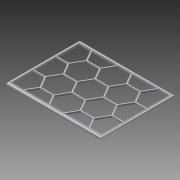
# Autodesk Inventor part: plate
Saved by Autodesk Inventor 2014 SP1 (Build 180222100, 222)
## iProperties
Created: 2016-09-05
Part Number: plate
Material: ABS Plastic
Document SubType Name: Modeling
Designer: tguillod
Density: 1.06 g/cm^3
Appearance: Smooth - White
Author: tguillod
Autodesk Inventor part; units mm, degrees
ref_plane "YZ Plane" through (0, 0, 0) normal (1, 0, 0) x (0, 1, 0)
ref_plane "XZ Plane" through (0, 0, 0) normal (0, 1, 0) x (-1, 0, 0)
ref_plane "XY Plane" through (0, 0, 0) normal (0, 0, 1) x (1, 0, 0)
sketch "Sketch1" plane through (0, 0, 0) normal (0, 0, 1) x (1, 0, 0)
  line L0 (0, 0) -> (183.5, 0)
  line L1 (183.5, 0) -> (183.5, 143)
  line L2 (183.5, 143) -> (0, 143)
  line L3 (0, 143) -> (0, 0)
  dimension "d0" = 183.5
  dimension "d1" = 143
  constraints: 8 end point, 2 parallel, 1 horizontal, 1 perpendicular
  measures "d0" distance of L1.end L2.end
  measures "d1" distance of L0.end L1.end
extrude "Extrusion1" add sketch "Sketch1" along normal blind 3
sketch "Sketch12" plane through (0, 0, 3) normal (0, 0, 1) x (1, 0, 0)
  line L0 (0, 0) -> (183.5, 0) projected
  line L1 (183.5, 0) -> (183.5, 143) projected
  line L2 (183.5, 143) -> (0, 143) projected
  line L3 (0, 143) -> (0, 0) projected
  line L4 (3, 5) -> (4, 5)
  line L5 (4, 5) -> (4, 140)
  line L6 (4, 140) -> (3, 140)
  line L7 (3, 140) -> (3, 5)
  line L8 (4, 140) -> (179.5, 140)
  line L9 (179.5, 140) -> (179.5, 139)
  line L10 (179.5, 139) -> (4, 139)
  line L11 (4, 139) -> (4, 140)
  line L12 (179.5, 140) -> (180.5, 140)
  line L13 (180.5, 140) -> (180.5, 5)
  line L14 (180.5, 5) -> (179.5, 5)
  line L15 (179.5, 5) -> (179.5, 140)
  dimension "d77" = 3
  dimension "d78" = 1
  dimension "d79" = 5
  dimension "d80" = 3
  dimension "d81" = 1
  dimension "d82" = 3
  dimension "d83" = 1
  constraints: 24 end point, 6 parallel, 3 horizontal, 3 perpendicular, 1 collinear
  measures "d77" distance between parallel lines of L3 L7
  measures "d78" distance of L4.start L4.end
  measures "d79" distance between parallel lines of L0 L4
  measures "d80" distance between parallel lines of L2 L8
  measures "d81" distance between parallel lines of L8 L10
  measures "d82" distance between parallel lines of L1 L13
  measures "d83" distance between parallel lines of L13 L15
extrude "Extrusion7" add sketch "Sketch12" along normal blind 1 contours L7 L6 L5 L4 | L5 L8 L9 L10 | L9 L12 L13 L14 L15
sketch "Sketch13" plane through (0, 0, 3) normal (0, 0, 1) x (1, 0, 0)
  line L0 (4, 139) -> (179.5, 139)
  line L1 (179.5, 139) -> (179.5, 5)
  line L2 (179.5, 5) -> (4, 5)
  line L3 (4, 5) -> (4, 139)
  line L4 (91.75, 139) -> (91.75, 5) construction
  line L5 (179.5, 72) -> (4, 72) construction
  line L6 (104.163, 50.5) -> (79.337, 50.5)
  line L7 (79.337, 50.5) -> (66.9239, 72)
  line L8 (66.9239, 72) -> (79.337, 93.5)
  line L9 (79.337, 93.5) -> (104.163, 93.5)
  line L10 (104.163, 93.5) -> (116.5761, 72)
  line L11 (116.5761, 72) -> (104.163, 50.5)
  line L12 (105.3177, 48.5) -> (78.1823, 48.5)
  line L13 (78.1823, 48.5) -> (64.6145, 72)
  line L14 (64.6145, 72) -> (78.1823, 95.5)
  line L15 (78.1823, 95.5) -> (105.3177, 95.5)
  line L16 (105.3177, 95.5) -> (118.8855, 72)
  line L17 (118.8855, 72) -> (105.3177, 48.5)
  line L18 (4, 139) -> (179.5, 139) projected
  line L19 (105.3177, 93.5) -> (78.1823, 93.5)
  line L20 (78.1823, 93.5) -> (64.6145, 117)
  line L21 (64.6145, 117) -> (78.1823, 140.5)
  line L22 (78.1823, 140.5) -> (105.3177, 140.5)
  line L23 (105.3177, 140.5) -> (118.8855, 117)
  line L24 (118.8855, 117) -> (105.3177, 93.5)
  line L25 (104.163, 95.5) -> (79.337, 95.5)
  line L26 (79.337, 95.5) -> (66.9239, 117)
  line L27 (66.9239, 117) -> (79.337, 138.5)
  line L28 (79.337, 138.5) -> (104.163, 138.5)
  line L29 (104.163, 138.5) -> (116.5761, 117)
  line L30 (116.5761, 117) -> (104.163, 95.5)
  line L31 (104.163, 5.5) -> (79.337, 5.5)
  line L32 (79.337, 5.5) -> (66.9239, 27)
  line L33 (66.9239, 27) -> (79.337, 48.5)
  line L34 (79.337, 48.5) -> (104.163, 48.5)
  line L35 (104.163, 48.5) -> (116.5761, 27)
  line L36 (116.5761, 27) -> (104.163, 5.5)
  line L37 (105.3177, 3.5) -> (78.1823, 3.5)
  line L38 (78.1823, 3.5) -> (64.6145, 27)
  line L39 (64.6145, 27) -> (78.1823, 50.5)
  line L40 (78.1823, 50.5) -> (105.3177, 50.5)
  line L41 (105.3177, 50.5) -> (118.8855, 27)
  line L42 (118.8855, 27) -> (105.3177, 3.5)
  line L43 (143.1342, 73) -> (118.3081, 73)
  line L44 (118.3081, 73) -> (105.8951, 94.5)
  line L45 (105.8951, 94.5) -> (118.3081, 116)
  line L46 (118.3081, 116) -> (143.1342, 116)
  line L47 (143.1342, 116) -> (155.5472, 94.5)
  line L48 (155.5472, 94.5) -> (143.1342, 73)
  line L49 (144.2889, 71) -> (117.1534, 71)
  line L50 (117.1534, 71) -> (103.5857, 94.5)
  line L51 (103.5857, 94.5) -> (117.1534, 118)
  line L52 (117.1534, 118) -> (144.2889, 118)
  line L53 (144.2889, 118) -> (157.8566, 94.5)
  line L54 (157.8566, 94.5) -> (144.2889, 71)
  line L55 (39.2111, 163) -> (66.3466, 163)
  line L56 (40.3658, 161) -> (65.1919, 161)
  line L57 (25.6434, 139.5) -> (39.2111, 163)
  line L58 (27.9528, 139.5) -> (40.3658, 161)
  line L59 (40.3658, 118) -> (27.9528, 139.5)
  line L60 (39.2111, 116) -> (25.6434, 139.5)
  line L61 (66.3466, 116) -> (39.2111, 116)
  line L62 (65.1919, 161) -> (77.6049, 139.5)
  line L63 (66.3466, 163) -> (79.9143, 139.5)
  line L64 (77.6049, 139.5) -> (65.1919, 118)
  line L65 (79.9143, 139.5) -> (66.3466, 116)
  line L66 (65.1919, 118) -> (40.3658, 118)
  line L67 (142.5568, 72) -> (156.1246, 95.5)
  line L68 (156.1246, 48.5) -> (142.5568, 72)
  line L69 (157.2793, 50.5) -> (144.8662, 72)
  line L70 (144.8662, 72) -> (157.2793, 93.5)
  line L71 (157.2793, 93.5) -> (182.1053, 93.5)
  line L72 (182.1053, 50.5) -> (157.2793, 50.5)
  line L73 (183.26, 48.5) -> (156.1246, 48.5)
  line L74 (156.1246, 95.5) -> (183.26, 95.5)
  line L75 (194.5183, 72) -> (182.1053, 50.5)
  line L76 (196.8277, 72) -> (183.26, 48.5)
  line L77 (182.1053, 93.5) -> (194.5183, 72)
  line L78 (183.26, 95.5) -> (196.8277, 72)
  line L79 (25.6434, 49.5) -> (39.2111, 73)
  line L80 (39.2111, 26) -> (25.6434, 49.5)
  line L81 (40.3658, 28) -> (27.9528, 49.5)
  line L82 (27.9528, 49.5) -> (40.3658, 71)
  line L83 (40.3658, 71) -> (65.1919, 71)
  line L84 (65.1919, 28) -> (40.3658, 28)
  line L85 (66.3466, 26) -> (39.2111, 26)
  line L86 (39.2111, 73) -> (66.3466, 73)
  line L87 (77.6049, 49.5) -> (65.1919, 28)
  line L88 (79.9143, 49.5) -> (66.3466, 26)
  line L89 (65.1919, 71) -> (77.6049, 49.5)
  line L90 (66.3466, 73) -> (79.9143, 49.5)
  line L91 (-13.3277, 72) -> (0.24, 95.5)
  line L92 (-11.0183, 72) -> (1.3947, 93.5)
  line L93 (0.24, 48.5) -> (-13.3277, 72)
  line L94 (1.3947, 50.5) -> (-11.0183, 72)
  line L95 (1.3947, 93.5) -> (26.2207, 93.5)
  line L96 (26.2207, 50.5) -> (1.3947, 50.5)
  line L97 (27.3754, 48.5) -> (0.24, 48.5)
  line L98 (0.24, 95.5) -> (27.3754, 95.5)
  line L99 (38.6338, 72) -> (26.2207, 50.5)
  line L100 (40.9432, 72) -> (27.3754, 48.5)
  line L101 (26.2207, 93.5) -> (38.6338, 72)
  line L102 (27.3754, 95.5) -> (40.9432, 72)
  line L103 (25.6434, 94.5) -> (39.2111, 118)
  line L104 (39.2111, 71) -> (25.6434, 94.5)
  line L105 (40.3658, 73) -> (27.9528, 94.5)
  line L106 (27.9528, 94.5) -> (40.3658, 116)
  line L107 (40.3658, 116) -> (65.1919, 116)
  line L108 (65.1919, 73) -> (40.3658, 73)
  line L109 (66.3466, 71) -> (39.2111, 71)
  line L110 (39.2111, 118) -> (66.3466, 118)
  line L111 (77.6049, 94.5) -> (65.1919, 73)
  line L112 (79.9143, 94.5) -> (66.3466, 71)
  line L113 (65.1919, 116) -> (77.6049, 94.5)
  line L114 (66.3466, 118) -> (79.9143, 94.5)
  line L115 (117.1534, 26) -> (103.5857, 49.5)
  line L116 (118.3081, 28) -> (105.8951, 49.5)
  line L117 (105.8951, 49.5) -> (118.3081, 71)
  line L118 (143.1342, 28) -> (118.3081, 28)
  line L119 (144.2889, 26) -> (117.1534, 26)
  line L120 (155.5472, 49.5) -> (143.1342, 28)
  line L121 (157.8566, 49.5) -> (144.2889, 26)
  line L122 (118.3081, 71) -> (143.1342, 71)
  line L123 (117.1534, 73) -> (144.2889, 73)
  line L124 (143.1342, 71) -> (155.5472, 49.5)
  line L125 (103.5857, 49.5) -> (117.1534, 73)
  line L126 (144.2889, 73) -> (157.8566, 49.5)
  line L127 (-13.3277, 117) -> (0.24, 140.5)
  line L128 (0.24, 93.5) -> (-13.3277, 117)
  line L129 (1.3947, 95.5) -> (-11.0183, 117)
  line L130 (-11.0183, 117) -> (1.3947, 138.5)
  line L131 (1.3947, 138.5) -> (26.2207, 138.5)
  line L132 (26.2207, 95.5) -> (1.3947, 95.5)
  line L133 (27.3754, 93.5) -> (0.24, 93.5)
  line L134 (0.24, 140.5) -> (27.3754, 140.5)
  line L135 (38.6338, 117) -> (26.2207, 95.5)
  line L136 (40.9432, 117) -> (27.3754, 93.5)
  line L137 (26.2207, 138.5) -> (38.6338, 117)
  line L138 (27.3754, 140.5) -> (40.9432, 117)
  line L139 (103.5857, 139.5) -> (117.1534, 163)
  line L140 (117.1534, 116) -> (103.5857, 139.5)
  line L141 (118.3081, 118) -> (105.8951, 139.5)
  line L142 (105.8951, 139.5) -> (118.3081, 161)
  line L143 (118.3081, 161) -> (143.1342, 161)
  line L144 (143.1342, 118) -> (118.3081, 118)
  line L145 (144.2889, 116) -> (117.1534, 116)
  line L146 (117.1534, 163) -> (144.2889, 163)
  line L147 (155.5472, 139.5) -> (143.1342, 118)
  line L148 (157.8566, 139.5) -> (144.2889, 116)
  line L149 (143.1342, 161) -> (155.5472, 139.5)
  line L150 (144.2889, 163) -> (157.8566, 139.5)
  line L151 (142.5568, 27) -> (156.1246, 50.5)
  line L152 (156.1246, 3.5) -> (142.5568, 27)
  line L153 (157.2793, 5.5) -> (144.8662, 27)
  line L154 (144.8662, 27) -> (157.2793, 48.5)
  line L155 (157.2793, 48.5) -> (182.1053, 48.5)
  line L156 (182.1053, 5.5) -> (157.2793, 5.5)
  line L157 (183.26, 3.5) -> (156.1246, 3.5)
  line L158 (194.5183, 27) -> (182.1053, 5.5)
  line L159 (196.8277, 27) -> (183.26, 3.5)
  line L160 (156.1246, 50.5) -> (183.26, 50.5)
  line L161 (182.1053, 48.5) -> (194.5183, 27)
  line L162 (183.26, 50.5) -> (196.8277, 27)
  line L163 (142.5568, 117) -> (156.1246, 140.5)
  line L164 (156.1246, 93.5) -> (142.5568, 117)
  line L165 (157.2793, 95.5) -> (144.8662, 117)
  line L166 (144.8662, 117) -> (157.2793, 138.5)
  line L167 (157.2793, 138.5) -> (182.1053, 138.5)
  line L168 (182.1053, 95.5) -> (157.2793, 95.5)
  line L169 (183.26, 93.5) -> (156.1246, 93.5)
  line L170 (194.5183, 117) -> (182.1053, 95.5)
  line L171 (196.8277, 117) -> (183.26, 93.5)
  line L172 (156.1246, 140.5) -> (183.26, 140.5)
  line L173 (182.1053, 138.5) -> (194.5183, 117)
  line L174 (183.26, 140.5) -> (196.8277, 117)
  line L175 (103.5857, 4.5) -> (117.1534, 28)
  line L176 (118.3081, 26) -> (143.1342, 26)
  line L177 (105.8951, 4.5) -> (118.3081, 26)
  line L178 (118.3081, -17) -> (105.8951, 4.5)
  line L179 (117.1534, -19) -> (103.5857, 4.5)
  line L180 (143.1342, 26) -> (155.5472, 4.5)
  line L181 (144.2889, 28) -> (157.8566, 4.5)
  line L182 (143.1342, -17) -> (118.3081, -17)
  line L183 (155.5472, 4.5) -> (143.1342, -17)
  line L184 (157.8566, 4.5) -> (144.2889, -19)
  line L185 (144.2889, -19) -> (117.1534, -19)
  line L186 (117.1534, 28) -> (144.2889, 28)
  line L187 (-13.3277, 27) -> (0.24, 50.5)
  line L188 (0.24, 3.5) -> (-13.3277, 27)
  line L189 (1.3947, 5.5) -> (-11.0183, 27)
  line L190 (-11.0183, 27) -> (1.3947, 48.5)
  line L191 (1.3947, 48.5) -> (26.2207, 48.5)
  line L192 (26.2207, 5.5) -> (1.3947, 5.5)
  line L193 (27.3754, 3.5) -> (0.24, 3.5)
  line L194 (0.24, 50.5) -> (27.3754, 50.5)
  line L195 (38.6338, 27) -> (26.2207, 5.5)
  line L196 (40.9432, 27) -> (27.3754, 3.5)
  line L197 (26.2207, 48.5) -> (38.6338, 27)
  line L198 (27.3754, 50.5) -> (40.9432, 27)
  line L199 (25.6434, 4.5) -> (39.2111, 28)
  line L200 (39.2111, -19) -> (25.6434, 4.5)
  line L201 (40.3658, -17) -> (27.9528, 4.5)
  line L202 (27.9528, 4.5) -> (40.3658, 26)
  line L203 (40.3658, 26) -> (65.1919, 26)
  line L204 (65.1919, -17) -> (40.3658, -17)
  line L205 (66.3466, -19) -> (39.2111, -19)
  line L206 (77.6049, 4.5) -> (65.1919, -17)
  line L207 (79.9143, 4.5) -> (66.3466, -19)
  line L208 (39.2111, 28) -> (66.3466, 28)
  line L209 (65.1919, 26) -> (77.6049, 4.5)
  line L210 (66.3466, 28) -> (79.9143, 4.5)
  point P0 (91.75, 72)
  point P1 (91.75, 72)
  point P2 (91.75, 117)
  point P3 (91.75, 117)
  point P4 (91.75, 27)
  point P5 (91.75, 27)
  point P6 (130.7211, 94.5)
  point P7 (130.7211, 94.5)
  point P8 (52.7789, 139.5)
  point P9 (52.7789, 139.5)
  point P10 (169.6923, 72)
  point P11 (169.6923, 72)
  point P12 (52.7789, 49.5)
  point P13 (52.7789, 49.5)
  point P14 (13.8077, 72)
  point P15 (13.8077, 72)
  point P16 (52.7789, 94.5)
  point P17 (52.7789, 94.5)
  point P18 (130.7211, 49.5)
  point P19 (130.7211, 49.5)
  point P20 (13.8077, 117)
  point P21 (13.8077, 117)
  point P22 (130.7211, 139.5)
  point P23 (130.7211, 139.5)
  point P24 (169.6923, 27)
  point P25 (169.6923, 27)
  point P26 (169.6923, 117)
  point P27 (169.6923, 117)
  point P28 (130.7211, 4.5)
  point P29 (130.7211, 4.5)
  point P30 (13.8077, 27)
  point P31 (13.8077, 27)
  point P32 (52.7789, 4.5)
  point P33 (52.7789, 4.5)
  dimension "d86" = 2
  dimension "d88" = 43
  dimension "d89" = 2
  dimension "d90" = 43
  dimension "d93" = 43
  dimension "d94" = 2
  dimension "d95" = 43
  dimension "d96" = 2
  dimension "d97" = 43
  dimension "d98" = 2
  dimension "d99" = 43
  dimension "d100" = 2
  dimension "d101" = 43
  dimension "d102" = 2
  dimension "d103" = 43
  dimension "d104" = 2
  dimension "d105" = 43
  dimension "d106" = 2
  dimension "d107" = 43
  dimension "d108" = 2
  dimension "d109" = 43
  dimension "d110" = 2
  dimension "d111" = 43
  dimension "d112" = 2
  dimension "d113" = 43
  dimension "d114" = 2
  dimension "d115" = 43
  dimension "d116" = 2
  dimension "d117" = 43
  dimension "d118" = 2
  dimension "d119" = 43
  dimension "d120" = 2
  dimension "d121" = 43
  dimension "d122" = 2
  constraints: 420 end point, 30 collinear, 17 coincident, 8 parallel, 5 midpoint, 2 point on line, 1 horizontal, 1 perpendicular, 442 other
  measures "d86" distance between parallel lines of L15 L9
  measures "d88" distance between parallel lines of L6 L9
  measures "d89" distance between parallel lines of L22 L28
  measures "d90" distance between parallel lines of L25 L28
  measures "d93" distance between parallel lines of L31 L34
  measures "d94" distance between parallel lines of L40 L34
  measures "d95" distance between parallel lines of L43 L46
  measures "d96" distance between parallel lines of L52 L46
  measures "d97" distance between parallel lines of L66 L56
  measures "d98" distance between parallel lines of L55 L56
  measures "d99" distance between parallel lines of L72 L71
  measures "d100" distance between parallel lines of L74 L71
  measures "d101" distance between parallel lines of L84 L83
  measures "d102" distance between parallel lines of L86 L83
  measures "d103" distance between parallel lines of L96 L95
  measures "d104" distance between parallel lines of L98 L95
  measures "d105" distance between parallel lines of L108 L107
  measures "d106" distance between parallel lines of L110 L107
  measures "d107" distance between parallel lines of L118 L122
  measures "d108" distance between parallel lines of L123 L122
  measures "d109" distance between parallel lines of L132 L131
  measures "d110" distance between parallel lines of L134 L131
  measures "d111" distance between parallel lines of L144 L143
  measures "d112" distance between parallel lines of L146 L143
  measures "d113" distance between parallel lines of L156 L155
  measures "d114" distance between parallel lines of L160 L155
  measures "d115" distance between parallel lines of L168 L167
  measures "d116" distance between parallel lines of L172 L167
  measures "d117" distance between parallel lines of L182 L176
  measures "d118" distance between parallel lines of L186 L176
  measures "d119" distance between parallel lines of L192 L191
  measures "d120" distance between parallel lines of L194 L191
  measures "d121" distance between parallel lines of L204 L203
  measures "d122" distance between parallel lines of L208 L203
extrude "Extrusion9" cut sketch "Sketch13" against normal blind 10 contours L131 L60 L103 L98 L3 | L3 L98 L129 L130 L131 | L59 L58 L56 L62 L21 L0 | L0 L21 L66 L59 | L95 L101 L79 L96 L3 | L3 L96 L94 L92 L95 | L28 L29 L30 L15 L26 L27 | L61 L20 L14 L86 L102 L106 | L97 L80 L195 L192 L3 | L3 L192 L189 L190 L97 | L23 L142 L143 L149 L147 L0 | L0 L147 L52 L23 | L82 L83 L13 L39 L84 L81 | L167 L1 L74 L53 L148 | L46 L47 L48 L43 L16 L24 | L9 L10 L11 L6 L7 L8 | L196 L85 L38 L2 | L2 L38 L206 L204 L201 L196 | L167 L173 L170 L74 L1 | L33 L12 L35 L36 L31 L32 | L71 L77 L75 L72 L1 | L1 L72 L69 L54 L71 | L49 L68 L120 L118 L41 L17 | L42 L119 L152 L2 | L2 L152 L183 L182 L178 L42 | L73 L161 L158 L156 L1 | L1 L156 L153 L121 L73
sketch "Sketch15" plane through (0, 0, 0) normal (0, 0, -1) x (-1, 0, 0)
  line L0 (-152.9491, 0) -> (-183.5, 0) projected
  line L1 (0, 0) -> (-30.5509, 0) projected
  line L2 (-183.5, 143) -> (-179.5, 143)
  line L3 (-179.5, 143) -> (-179.5, 0)
  line L4 (-179.5, 0) -> (-183.5, 0)
  line L5 (-183.5, 0) -> (-183.5, 143)
  line L6 (0, 143) -> (-4, 143)
  line L7 (-4, 143) -> (-4, 0)
  line L8 (-4, 0) -> (0, 0)
  line L9 (0, 0) -> (0, 143)
  line L10 (-179.5, 143) -> (-4, 143)
  line L11 (-4, 143) -> (-4, 138.5)
  line L12 (-4, 138.5) -> (-179.5, 138.5)
  line L13 (-179.5, 138.5) -> (-179.5, 143)
  line L14 (-179.5, 0) -> (-4, 0)
  line L15 (-4, 0) -> (-4, 6)
  line L16 (-4, 6) -> (-179.5, 6)
  line L17 (-179.5, 6) -> (-179.5, 0)
  dimension "d129" = 4.5
  dimension "d130" = 4
  dimension "d131" = 4
  dimension "d132" = 6
  constraints: 32 end point, 8 parallel, 4 horizontal, 4 perpendicular, 4 point on line
  measures "d129" distance between parallel lines of L10 L12
  measures "d130" distance between parallel lines of L5 L3
  measures "d131" distance between parallel lines of L7 L9
  measures "d132" distance between parallel lines of L16 L14
extrude "Extrusion10" add sketch "Sketch15" against normal blind 3 contours L0 L3 L16 L7 L1 L14 | L0 L5 L2 L3 | L7 L6 L9 L1 | L3 L10 L7 L12
sketch "Sketch16" plane through (0, 0, 3) normal (0, 0, 1) x (1, 0, 0)
  line L0 (4, 5) -> (179.5, 5)
  line L1 (179.5, 5) -> (179.5, 6)
  line L2 (179.5, 6) -> (4, 6)
  line L3 (4, 6) -> (4, 5)
  constraints: 8 end point, 2 parallel, 1 horizontal, 1 perpendicular
extrude "Extrusion11" add sketch "Sketch16" along normal blind 1
body "Solid1"
